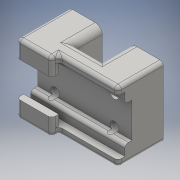
# Autodesk Inventor part: NrfMount
Saved by Autodesk Inventor 2016 (Build 200138000, 138)
## iProperties
Created: 2026-03-25
Part Number: NrfMount
Material: Generic
Document SubType Name: Modeling
Designer: Steve
Density: 1 g/cm^3
Appearance: Default
Author: Steve
Autodesk Inventor part; units mm, degrees
ref_plane "YZ Plane" through (0, 0, 0) normal (1, 0, 0) x (0, 1, 0)
ref_plane "XZ Plane" through (0, 0, 0) normal (0, 1, 0) x (-1, 0, 0)
ref_plane "XY Plane" through (0, 0, 0) normal (0, 0, 1) x (1, 0, 0)
sketch "Sketch1" plane through (0, 0, 0) normal (0, 1, 0) x (-1, 0, 0)
  line L0 (7.2077, 13.5916) -> (-19.7923, 13.5916)
  line L1 (-19.7923, 13.5916) -> (-19.7923, -6.4084)
  line L2 (-19.7923, -6.4084) -> (7.2077, -6.4084)
  line L3 (7.2077, -6.4084) -> (7.2077, 13.5916)
  circle A0 centre (2.2077, 7.5916) radius 1.25
  circle A1 centre (2.2077, -0.4084) radius 1.25
  circle A2 centre (-14.7923, 7.5916) radius 1.25
  circle A3 centre (-14.7923, -0.4084) radius 1.25
  point P0 (0, 0)
  dimension "d0" = 20
  dimension "d1" = 27
  dimension "d5" = 5
  dimension "d9" = 5
  dimension "d14" = 5
  dimension "d15" = 5
  dimension "d20" = 8
  dimension "d21" = 8
  dimension "d22" = 17
  dimension "d23" = 17
  dimension "d24" = 2.5
  dimension "d25" = 2.5
  dimension "d26" = 2.5
  dimension "d27" = 2.5
  dimension "d43" = 6
  dimension "d44" = 6
  dimension "d45" = 6
  dimension "d46" = 6
  constraints: 8 end point, 4 centre point, 4 coincident, 2 parallel, 1 horizontal, 1 perpendicular
  measures "d0" distance of L2.end L0.start
  measures "d1" distance of L1.end L2.end
  measures "d5" distance from line of L3 point (2.208, 7.592)
  measures "d9" distance from line of L3 point (2.208, -0.408)
  measures "d14" distance from line of L1 point (-14.792, -0.408)
  measures "d15" distance from line of L1 point (-14.792, 7.592)
  measures "d20" distance of point (2.208, -0.408) point (2.208, 7.592)
  measures "d21" distance of point (-14.792, -0.408) point (-14.792, 7.592)
  measures "d22" distance of point (2.208, -0.408) point (-14.792, -0.408)
  measures "d23" distance of point (-14.792, 7.592) point (2.208, 7.592)
  measures "d24" diameter of A0
  measures "d25" diameter of A1
  measures "d26" diameter of A2
  measures "d27" diameter of A3
  measures "d43" distance from line of L0 point (2.208, 7.592)
  measures "d44" distance from line of L2 point (2.208, -0.408)
  measures "d45" distance from line of L0 point (-14.792, 7.592)
  measures "d46" distance from line of L2 point (-14.792, -0.408)
extrude "Extrusion4" add sketch "Sketch1" along normal blind 2 contours A0 | A1 | A2 | A3
extrude "Extrusion1" add sketch "Sketch1" along normal blind 13 separate body
sketch "Sketch2" plane through (0, 0, 0) normal (0, -1, 0) x (1, 0, 0)
  line L0 (-7.2077, -6.4084) -> (-7.2077, 13.5916) projected
  line L1 (-7.2077, -1.4084) -> (19.7923, -1.4084)
  line L2 (19.7923, -1.4084) -> (19.7923, 8.5916)
  line L3 (19.7923, 8.5916) -> (-7.2077, 8.5916)
  line L4 (-7.2077, 8.5916) -> (-7.2077, -1.4084)
  line L5 (19.7923, -6.4084) -> (-7.2077, -6.4084) projected
  point P0 (0, 0)
  dimension "d32" = 27
  dimension "d33" = 10
  dimension "d34" = 5
  constraints: 8 end point, 2 parallel, 1 horizontal, 1 perpendicular, 1 point on line
  measures "d32" distance of L3.end L2.end
  measures "d33" distance of L2.end L1.end
  measures "d34" distance between parallel lines of L5 L1
extrude "Extrusion3" cut sketch "Sketch2" against normal blind 4
sketch "Sketch4" plane through (0, 0, 0) normal (0, -1, 0) x (1, 0, 0)
  line L0 (19.7923, 11.5916) -> (-7.2077, 11.5916)
  line L1 (-7.2077, 11.5916) -> (-7.2077, -4.4084)
  line L2 (-7.2077, -4.4084) -> (19.7923, -4.4084)
  line L3 (19.7923, -4.4084) -> (19.7923, 11.5916)
  line L4 (-7.2077, 13.5916) -> (19.7923, 13.5916) projected
  line L5 (-7.2077, -1.4084) -> (-7.2077, 8.5916) projected
  line L6 (19.7923, 13.5916) -> (19.7923, -6.4084) projected
  point P0 (0, 0)
  dimension "d47" = 16
  dimension "d50" = 2
  dimension "d51" = 0
  dimension "d52" = 0
  constraints: 8 end point, 2 parallel, 1 horizontal, 1 perpendicular
  measures "d47" distance of L2.end L0.start
  measures "d50" distance between parallel lines of L4 L0
  measures "d51" distance between parallel lines of L5 L1
  measures "d52" distance between parallel lines of L6 L3
extrude "Extrusion7" cut sketch "Sketch4" against normal blind 2
sketch "Sketch6" plane through (19.7923, 0, -6.4084) normal (0, 0, -1) x (-1, 0, 0)
  line L0 (0, 13) -> (27, 13) projected
  line L1 (17.5, 13) -> (9.5, 13)
  line L2 (9.5, 13) -> (9.5, 5)
  line L3 (9.5, 5) -> (17.5, 5)
  line L4 (17.5, 5) -> (17.5, 13)
  line L5 (0, 0) -> (0, 13) projected
  line L6 (27, 0) -> (27, 13) projected
  point P0 (19.7923, 0)
  dimension "d65" = 8
  dimension "d66" = 8
  dimension "d67" = 9.5
  dimension "d68" = 9.5
  constraints: 8 end point, 2 parallel, 1 horizontal, 1 perpendicular, 1 point on line
  measures "d65" distance of L3.end L2.end
  measures "d66" distance of L2.end L1.end
  measures "d67" distance between parallel lines of L5 L2
  measures "d68" distance between parallel lines of L6 L4
extrude "Extrusion10" cut sketch "Sketch6" against normal through all
sketch "Sketch7" plane through (-7.2077, 0, 13.5916) normal (-1, 0, 0) x (0, 0, 1)
  line L0 (-2, 0) -> (0, 0) projected
  line L1 (0, 0) -> (-5, 0)
  line L2 (-5, 0) -> (-5, -2)
  line L3 (-5, -2) -> (0, -2)
  line L4 (0, -2) -> (0, 0)
  line L5 (-20, 0) -> (-20, 13) projected
  line L6 (-20, 0) -> (-15, 0)
  line L7 (-15, 0) -> (-15, -2)
  line L8 (-15, -2) -> (-20, -2)
  line L9 (-20, -2) -> (-20, 0)
  point P0 (-13.5916, 0)
  dimension "d71" = 5
  dimension "d72" = 2
  dimension "d73" = 5
  dimension "d74" = 2
  constraints: 16 end point, 4 parallel, 2 horizontal, 2 perpendicular
  measures "d71" distance of L3.end L2.end
  measures "d72" distance of L2.end L1.end
  measures "d73" distance of L7.end L8.end
  measures "d74" distance of L6.end L7.end
extrude "Extrusion11" add sketch "Sketch7" against normal blind 10
fillet "Fillet3" radius 2 6 edges at (2.2923, 9, -6.4084) (6.2923, 5, -6.4084) (10.2923, 9, -6.4084) (10.2923, 9, 13.5916) (6.2923, 5, 13.5916) (2.2923, 9, 13.5916)
fillet "Fillet4" radius 1 4 edges at (11.2923, 0, -6.4084) (2.7923, -1, -6.4084) (-2.2077, -2, -6.4084) (2.7923, -2, -3.9084)
fillet "Fillet5" radius 1 8 edges at (2.4994, 0.2929, -6.1155) (2.7923, 0, -4.9084) (-7.2077, -1.7071, -6.1155) (-7.2077, 6, -6.4084) (-7.2077, -2, -3.4084) (19.7923, 0.2929, -6.1155) (19.7923, 0, -4.9084) (19.7923, 7, -6.4084)
fillet "Fillet6" radius 1 5 edges at (-2.2077, -2, 13.5916) (2.7923, -1, 13.5916) (11.2923, 0, 13.5916) (19.7923, 6.5, 13.5916) (-7.2077, 5.5, 13.5916)
fillet "Fillet7" radius 1 8 edges at (2.4994, -1.7071, 13.2988) (2.7923, -2, 10.5916) (2.4994, 0.2929, 13.2988) (2.7923, 0, 12.0916) (-6.9148, -1.7071, 13.2988) (-7.2077, -2, 10.5916) (19.7923, 0, 12.0916) (19.4994, 0.2929, 13.2988)
fillet "Fillet8" radius 1 2 edges at (6.2923, 2, 8.5916) (6.2923, 2, -1.4084)
body "Solid1"
